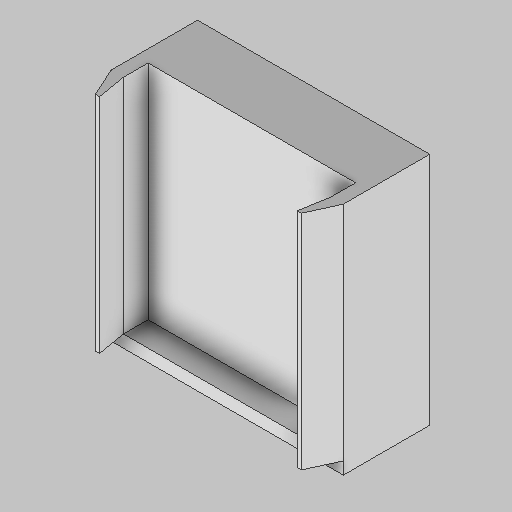
# Autodesk Inventor part: 2. ALARME
Saved by Autodesk Inventor 2025.2 (Build 292293000, 293)
## iProperties
Created: 2025-01-16
Part Number: 2. ALARME
Material: Genérico
Document SubType Name: Modeling
Designer: phmca
Density: 1 g/cm^3
Appearance: Padrão
Author: phmca
Autodesk Inventor part; units mm, degrees
ref_plane "YZ Plane" through (0, 0, 0) normal (1, 0, 0) x (0, 1, 0)
ref_plane "XZ Plane" through (0, 0, 0) normal (0, 1, 0) x (-1, 0, 0)
ref_plane "XY Plane" through (0, 0, 0) normal (0, 0, 1) x (1, 0, 0)
sketch "Esboço1" plane through (26.7, 48.5, -7.5) normal (0, 1, 0) x (-1, 0, 0)
  line L0 (0, 0) -> (28.2, 0) projected
  line L1 (0, 10.5) -> (0, 0) projected
  line L2 (1.6, 14) -> (0, 10.5) projected
  line L3 (2.1, 14) -> (1.6, 14) projected
  line L4 (1.5, 10.5) -> (2.1, 14) projected
  line L5 (26.1, 14) -> (26.7, 10.5) projected
  line L6 (26.6, 14) -> (26.1, 14) projected
  line L7 (28.2, 10.5) -> (26.6, 14) projected
  line L8 (28.2, 0) -> (28.2, 10.5) projected
  line L9 (26.7, 7.5) -> (1.5, 7.5) projected
  line L10 (1.5, 7.5) -> (1.5, 10.5) projected
  line L11 (26.7, 10.5) -> (26.7, 7.5) projected
extrude "Extrusão1" add sketch "Esboço1" against normal blind 27
sketch "Esboço2" plane through (25.2, 21.5, 3) normal (0, 0, 1) x (1, 0, 0)
  line L0 (1.5, 0) -> (-26.7, 0) projected
  line L1 (-26.7, -1.5) -> (1.5, -1.5) projected
  line L2 (1.5, -1.5) -> (1.5, 27) projected
  line L3 (-26.7, 27) -> (-26.7, -1.5) projected
  point P0 (-25.2, -21.5)
extrude "Extrusão2" add sketch "Esboço2" against normal up to surface (10.5 mm away)
